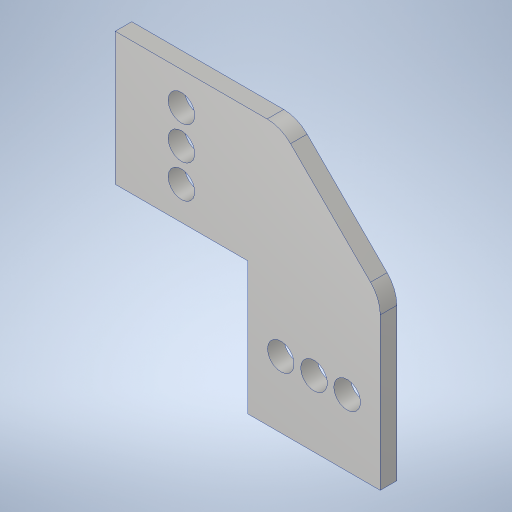
# Autodesk Inventor part: EL2-010
Saved by Autodesk Inventor 2023.4 (Build 274418000, 418)
## iProperties
Created: 2025-01-12
Part Number: EL2-010
Material: Aluminum 6061
Document SubType Name: Modeling
Designer: mavericks
Density: 2.7 g/cm^3
Appearance: Aluminum - Flat
Author: mavericks
Autodesk Inventor part; units mm, degrees
ref_plane "YZ Plane" through (0, 0, 0) normal (1, 0, 0) x (0, 1, 0)
ref_plane "XZ Plane" through (0, 0, 0) normal (0, 1, 0) x (-1, 0, 0)
ref_plane "XY Plane" through (0, 0, 0) normal (0, 0, 1) x (1, 0, 0)
sketch "Sketch1" plane through (0, 0, 0) normal (0, 0, 1) x (1, 0, 0)
  line L0 (0, 0) -> (25.4, 0) construction
  line L1 (25.4, 0) -> (25.4, 76.2) construction
  line L2 (25.4, 76.2) -> (0, 76.2) construction
  line L3 (0, 76.2) -> (0, 0) construction
  line L4 (25.4, 0) -> (101.6, 0) construction
  line L5 (101.6, 0) -> (101.6, -25.4) construction
  line L6 (101.6, -25.4) -> (25.4, -25.4) construction
  line L7 (25.4, -25.4) -> (25.4, 0) construction
  line L8 (25.4, 0) -> (0, 0)
  line L9 (0, 25.4) -> (0, 0)
  line L10 (0, 25.4) -> (50.8, 25.4)
  line L11 (50.8, 25.4) -> (50.8, -25.4)
  line L12 (25.4, -25.4) -> (50.8, -25.4)
  line L13 (25.4, -25.4) -> (25.4, 0)
  point P0 (12.7, 6.35)
  point P1 (12.7, 19.05)
  point P2 (12.7, 12.7)
  point P3 (12.7, 0)
  point P4 (31.75, -12.7)
  point P5 (38.1, -12.7)
  point P6 (44.45, -12.7)
  point P7 (25.4, -12.7)
  dimension "d0" = 25.4
  dimension "d1" = 76.2
  dimension "d2" = 76.2
  dimension "d3" = 25.4
  dimension "d4" = 31.75
  dimension "d5" = 6.35
  dimension "d6" = 6.35
  dimension "d7" = 6.35
  dimension "d8" = 6.35
  dimension "d9" = 31.75
  dimension "d10" = 25.4
  dimension "d11" = 25.4
  constraints: 28 end point, 4 parallel, 4 perpendicular, 3 collinear, 3 horizontal, 3 horizontal alignment, 3 vertical alignment, 2 midpoint, 2 point on line, 1 coincident
  measures "d0" distance of L2.end L1.end
  measures "d1" distance of L1.end L0.end
  measures "d2" distance of L5.end L6.end
  measures "d3" distance of L4.end L5.end
  measures "d4" vertical distance of L6.end point (12.7, 6.35)
  measures "d5" distance of point (12.7, 12.7) point (12.7, 6.35)
  measures "d6" distance of point (12.7, 19.05) point (12.7, 12.7)
  measures "d7" distance of point (38.1, -12.7) point (31.75, -12.7)
  measures "d8" distance of point (44.45, -12.7) point (38.1, -12.7)
  measures "d9" horizontal distance of point (0, 0) point (31.75, -12.7)
  measures "d10" distance between parallel lines of L11 L7
  measures "d11" distance between parallel lines of L8 L10
extrude "Extrusion1" add sketch "Sketch1" along normal blind 3.175
hole "Hole1" at (12.7, 6.35, 0) at (12.7, 19.05, 0) at (12.7, 12.7, 0) at (31.75, -12.7, 0) at (38.1, -12.7, 0) at (44.45, -12.7, 0) direction (0, 0, 1) diameter 5.1054 end through all clearance for "Flat Head Machine Screw (82)" size "#10" standard "Ansi Unified Screw Threads"
chamfer "Chamfer1" distance 19.05 angle 45 1 edges at (50.8, 25.4, 1.5875)
fillet "Fillet2" radius 6.35 2 edges at (31.75, 25.4, 1.5875) (50.8, 6.35, 1.5875)
equation "\"d6\" = d5"
equation "\"d10\" = d11"
body "Solid1"
